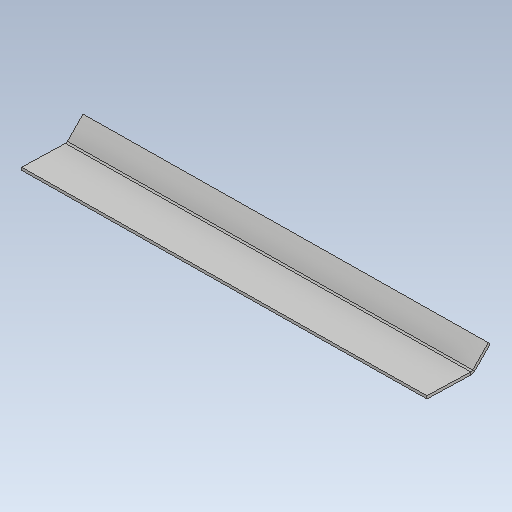
# Autodesk Inventor part: Skena
Saved by Autodesk Inventor 2021 (Build 250183000, 183)
## iProperties
Created: 2019-04-15
Part Number: Skena
Material: Generic
Document SubType Name: Sheet Metal
Designer: CASE-SMALL2
Density: 1 g/cm^3
Sheet Metal Rule: Default_mm
Appearance: Default
Flat Pattern Width: 7.55437 cm
Flat Pattern Length: 46 cm
Flat Pattern Area: 347.501 cm^2
Sheet Metal Width: 75,544 mm
Sheet Metal Length: 460,000 mm
Sheet Metal Area: 34750,092 mm^2
Author: CASE-SMALL2
Autodesk Inventor part; units mm, degrees
ref_plane "YZ Plane" through (0, 0, 0) normal (1, 0, 0) x (0, 1, 0)
ref_plane "XZ Plane" through (0, 0, 0) normal (0, 1, 0) x (-1, 0, 0)
sketch "Sketch3" plane through (230, 25, 3) normal (0, 0.7071068, 0.7071068) x (1, 0, 0)
  line L0 (0, 0) -> (-460, 0)
  line L1 (-460, 0) -> (-460, 27.12132)
  line L2 (-460, 27.12132) -> (0, 27.12132)
  line L3 (0, 27.12132) -> (0, 0)
  line L4 (0, 2.12132) -> (-460, 2.12132)
  line L5 (-460, -35.355339) -> (-460, 0)
  point P0 (-230, -15.556349)
  dimension "d4" = 25
  dimension "d5" = 0
  measures "d4" distance between parallel lines of L2 L4
  measures "d5" distance between parallel lines of L5 L1
sketch "Sketch1 outline for Plate1" plane through (0, 0, 0) normal (0, 0, 1) x (1, 0, 0)
  line L0 (-230, 25) -> (-230, -25)
  line L1 (230, 25) -> (-230, 25)
  line L2 (230, -25) -> (230, 25)
  line L3 (-230, -25) -> (230, -25)
extrude "Plate1" add sketch "Sketch1 outline for Plate1" along normal blind 3
sketch "Sketch1" plane through (0, 0, 0) normal (0, 0, 1) x (1, 0, 0)
  line L0 (-230, -25) -> (230, -25)
  line L1 (230, -25) -> (230, 25)
  line L2 (230, 25) -> (-230, 25)
  line L3 (-230, 25) -> (-230, -25)
  line L4 (-230, -25) -> (230, 25) construction
  line L5 (230, -25) -> (-230, 25) construction
  point P0 (0, 0)
  dimension "d0" = 460
  dimension "d1" = 50
  measures "d0" distance of L1.end L2.end
  measures "d1" distance of L2.end L0.start
ref_plane "Work Plane1" through (230, 25, 3) normal (0, 0.7071068, 0.7071068) x (1, 0, 0)
sketch "Sketch3 outline for Plate2" plane through (230, 25, 3) normal (0, 0.7071068, 0.7071068) x (1, 0, 0)
  line L0 (0, 0) -> (-460, 0)
  line L1 (-460, 0) -> (-460, 27.12132)
  line L2 (-460, 27.12132) -> (0, 27.12132)
  line L3 (0, 27.12132) -> (0, 2.12132)
  line L4 (0, 2.12132) -> (0, 0)
sheet face with bend "Face2" sketch "Sketch3 outline for Plate2" thickness 3 toward (0, -0.7071068, -0.7071068) bend radius 3
bend "Bend1"
equation "\"d2\" = Thickness"
equation "\"d6\" = BendRadius"
equation "\"d7\" = BendReliefWidth"
equation "\"d9\" = MinimumRemnant"
equation "\"d8\" = BendReliefDepth"
equation "\"d10\" = TransitionRadius"
equation "\"BendRadius\" = Thickness"
equation "\"BendReliefWidth\" = Thickness"
equation "\"BendReliefDepth\" = 0.5 * Thickness"
equation "\"CornerReliefSize\" = 4 * Thickness"
equation "\"MinimumRemnant\" = 2 * Thickness"
equation "\"TransitionRadius\" = BendRadius"
equation "\"JacobiRadiusSize\" = BendRadius"
equation "\"GapSize\" = Thickness"
equation "\"Thickness\" = 3"
body "Solid1"
